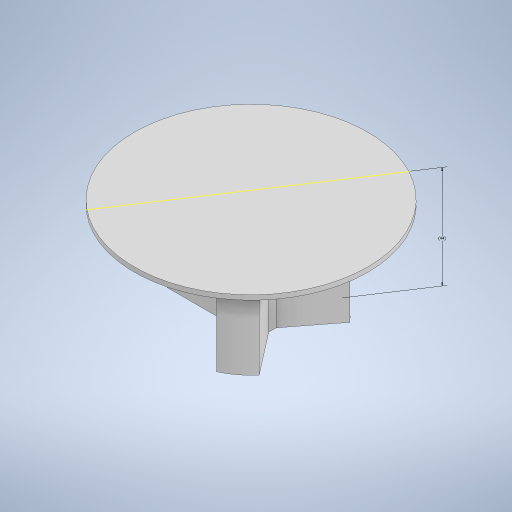
# Autodesk Inventor part: Peça1
Saved by Autodesk Inventor 2024.3 (Build 283343000, 343)
## iProperties
Created: 2024-12-05
Part Number: Peça1
Material: Genérico
Document SubType Name: Modeling
Designer: lostv
Density: 1 g/cm^3
Appearance: Padrão
Author: lostv
Autodesk Inventor part; units mm, degrees
ref_plane "YZ Plane" through (0, 0, 0) normal (1, 0, 0) x (0, 1, 0)
ref_plane "XZ Plane" through (0, 0, 0) normal (0, 1, 0) x (-1, 0, 0)
ref_plane "XY Plane" through (0, 0, 0) normal (0, 0, 1) x (1, 0, 0)
sketch "Esboço1" plane through (0, 0, 0) normal (0, 1, 0) x (-1, 0, 0)
  circle A0 centre (0, 0) radius 30
  line L0 (29.2563, 6.6384) -> (1.1855, 6.6384)
  line L1 (1.1855, 6.6384) -> (-12.4256, 27.3058)
  line L2 (-22.8619, 19.4251) -> (-7.7387, -0.1879)
  line L3 (29.9994, -0.1879) -> (-29.9994, -0.1879) construction
  line L4 (29.2563, -7.0142) -> (1.1855, -7.0142)
  line L5 (1.1855, -7.0142) -> (-12.4256, -27.6816)
  line L6 (-22.8619, -19.8009) -> (-7.7387, -0.1879)
  point P0 (29.2563, -6.6384)
  point P1 (-23.0884, -19.1553)
  point P2 (-22.7094, -19.6031)
  point P3 (29.1685, -7.0142)
  point P4 (-12.2347, -27.3918)
  dimension "d0" = 60
  constraints: 14 end point, 4 symmetric about line, 2 horizontal, 1 coincident, 9 other
extrude "Extrusão1" add sketch "Esboço1" along normal blind 42 contours A0 L4 L5 L6 L2 L1 L0
sketch "Esboço2" plane through (0, 42, 0) normal (0, 1, 0) x (1, 0, 0)
  circle A0 centre (0, 0) radius 50
  dimension "d3" = 100
  constraints: 1 centre point, 1 coincident
  measures "d3" diameter of A0
extrude "Extrusão2" add sketch "Esboço2" along normal blind 2
chamfer "Chanfro1" distance 2 angle 45 3 edges at (-1.1855, 21, -7.0142) (-1.1855, 21, 6.6384) (7.7387, 21, -0.1879)
sketch "Esboço3" plane through (12.2347, 0, -27.3918) normal (-0.8352, 0, -0.55) x (-0.55, 0, 0.8352)
  line L0 (23.1979, 0) -> (0.7435, 0) projected
  line L1 (79.6057, 44) -> (-20.3943, 44) projected
  point P0 (29.6057, 0)
  dimension "d10" = 44
  measures "d10" distance between parallel lines of L0 L1
